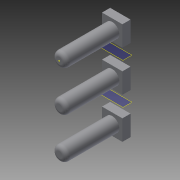
# Autodesk Inventor part: Part2
Saved by Autodesk Inventor 2014 SP1 (Build 180222100, 222)
## iProperties
Created: 2013-12-01
Part Number: Part2
Material: Generic
Document SubType Name: Modeling
Designer: Tim
Density: 1 g/cm^3
Appearance: Default
Author: Tim
Autodesk Inventor part; units mm, degrees
ref_plane "YZ Plane" through (0, 0, 0) normal (1, 0, 0) x (0, 1, 0)
ref_plane "XZ Plane" through (0, 0, 0) normal (0, 1, 0) x (-1, 0, 0)
ref_plane "XY Plane" through (0, 0, 0) normal (0, 0, 1) x (1, 0, 0)
sketch "Sketch1" plane through (0, 0, 0) normal (0, 1, 0) x (-1, 0, 0)
  circle A0 centre (0, 0) radius 1.75
  dimension "d1" = 3.5
  dimension "d5" = 0
  constraints: 1 centre point
  measures "d1" diameter of A0
  measures "d5" distance of point (0, 0) A0.centre
extrude "Extrusion1" add sketch "Sketch1" along normal blind 13
sketch "Sketch5" plane through (0, 13, 0) normal (0, 1, 0) x (1, 0, 0)
  circle A0 centre (0, 0) radius 1.75 projected
  line L0 (-2.5, -2.5) -> (2.5, -2.5)
  line L1 (2.5, -2.5) -> (2.5, 2.5)
  line L2 (2.5, 2.5) -> (-2.5, 2.5)
  line L3 (-2.5, 2.5) -> (-2.5, -2.5)
  line L4 (-2.5, -2.5) -> (2.5, 2.5) construction
  line L5 (2.5, -2.5) -> (-2.5, 2.5) construction
  dimension "d14" = 5
  dimension "d15" = 5
  constraints: 12 end point, 2 midpoint, 2 parallel, 1 horizontal, 1 perpendicular
  measures "d14" distance between parallel lines of L0 L2
  measures "d15" distance between parallel lines of L3 L1
extrude "Extrusion2" add sketch "Sketch5" along normal blind 2 contours A0 | L3 L2 L1 L0
sketch "Sketch6" plane through (0, 0, 0) normal (0, 1, 0) x (-1, 0, 0)
  point P0 (0, 0)
ref_plane "Work Plane1" through (2.5, 13, -5) normal (0, 0, -1) x (-1, 0, 0)
mirror "Mirror1" about plane through (2.5, 13, -5) normal (0, 0, -1)
ref_plane "Work Plane2" through (2.5, 13, -15) normal (0, 0, -1) x (-1, 0, 0)
mirror "Mirror2" about plane through (2.5, 13, -15) normal (0, 0, -1) of "Mirror1"
fillet "Fillet1" radius 1 3 edges at (1.75, 0, 0) (1.75, 0, -10) (1.75, 0, -20)
equation "\"d1\" = d0"
equation "\"d15\" = d14"
equation "\"d0\" = 3.5"
body "Solid1"
